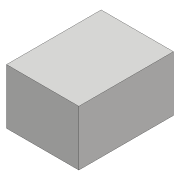
# Autodesk Inventor part: Деталь
Saved by Autodesk Inventor 2017 (Build 210142000, 142)
## iProperties
Part Number: Деталь
Material: Типовые
Document SubType Name: Modeling
Designer: Евтушенко
Density: 1 g/cm^3
Appearance: По умолчанию
Author: Евтушенко
Autodesk Inventor part; units mm, degrees
ref_plane "YZ Plane" through (0, 0, 0) normal (1, 0, 0) x (0, 1, 0)
ref_plane "XZ Plane" through (0, 0, 0) normal (0, 1, 0) x (-1, 0, 0)
ref_plane "XY Plane" through (0, 0, 0) normal (0, 0, 1) x (1, 0, 0)
sketch "Эскиз1" plane through (0, 0, 0) normal (0, 0, 1) x (1, 0, 0)
  line L0 (-340, -445) -> (340, -445)
  line L1 (340, -445) -> (340, 445)
  line L2 (340, 445) -> (-340, 445)
  line L3 (-340, 445) -> (-340, -445)
  line L4 (-340, -445) -> (340, 445) construction
  line L5 (340, -445) -> (-340, 445) construction
  point P0 (0, 0)
  dimension "d0" = 680
  dimension "d1" = 890
  constraints: 12 end point, 2 midpoint, 2 parallel, 1 horizontal, 1 perpendicular
  measures "d0" distance of L2.end L1.end
  measures "d1" distance of L1.end L0.end
extrude "Выдавливание1" add sketch "Эскиз1" along normal mid plane 520
